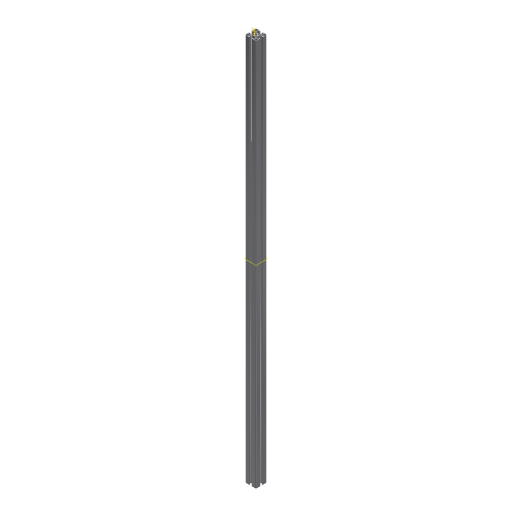
# Autodesk Inventor part: Profil-40x40x1200
Saved by Autodesk Inventor 2024.3 (Build 283343000, 343)
## iProperties
Created: 2012-07-12
Part Number: Profil-40x40x1200
Document SubType Name: Modeling
Designer: rd
Density: 2.7 g/cm^3
Material: Aluminium 6061
Appearance: Aluminium - poliert
Mass: 416.439 g
Surface Area: 1756.69 cm^2
Volume: 154.237 cm^3
Author: rd
Autodesk Inventor part; units mm, degrees
ref_plane "YZ Plane" through (0, 0, 0) normal (1, 0, 0) x (0, 1, 0)
ref_plane "XZ Plane" through (0, 0, 0) normal (0, 1, 0) x (-1, 0, 0)
sketch "Skizze1" plane through (0, 0, 0) normal (0, 0, 1) x (1, 0, 0)
  line L0 (4.8272, 8.2658) -> (6.2339, 9.6725)
  arc A0 (6.8957, 9.7126) -> (6.2339, 9.6725) centre (6.5874, 9.3189) ccw
  line L1 (6.8957, 9.7126) -> (7.2389, 9.4483)
  arc A1 (7.2389, 9.4483) -> (9.17, 8.8) centre (9.17, 12) ccw
  line L2 (9.17, 8.8) -> (12.7997, 8.8)
  arc A2 (13.2997, 8.3) -> (12.7997, 8.8) centre (12.7997, 8.3) ccw
  line L3 (13.2997, 8.3) -> (13.2997, 4)
  arc A3 (10.4997, 1.2) -> (13.2997, 4) centre (10.4997, 4) ccw
  line L4 (10.4997, 1.2) -> (6.1997, 1.2)
  arc A4 (5.6997, 1.7) -> (6.1997, 1.2) centre (6.1997, 1.7) ccw
  line L5 (5.6997, 1.7) -> (5.6997, 5.3296)
  arc A5 (5.6997, 5.3296) -> (5.0513, 7.2607) centre (2.4997, 5.3296) ccw
  line L6 (5.0513, 7.2607) -> (4.7871, 7.6039)
  arc A6 (4.8272, 8.2658) -> (4.7871, 7.6039) centre (5.1807, 7.9122) ccw
  line L7 (-15.8272, 31.7342) -> (-17.2339, 30.3275)
  arc A7 (-17.8957, 30.2874) -> (-17.2339, 30.3275) centre (-17.5874, 30.6811) ccw
  line L8 (-17.8957, 30.2874) -> (-18.2389, 30.5517)
  arc A8 (-18.2389, 30.5517) -> (-20.17, 31.2) centre (-20.17, 28) ccw
  line L9 (-20.17, 31.2) -> (-23.7997, 31.2)
  arc A9 (-24.2997, 31.7) -> (-23.7997, 31.2) centre (-23.7997, 31.7) ccw
  line L10 (-24.2997, 31.7) -> (-24.2997, 36)
  arc A10 (-21.4997, 38.8) -> (-24.2997, 36) centre (-21.4997, 36) ccw
  line L11 (-21.4997, 38.8) -> (-17.1997, 38.8)
  arc A11 (-16.6997, 38.3) -> (-17.1997, 38.8) centre (-17.1997, 38.3) ccw
  line L12 (-16.6997, 38.3) -> (-16.6997, 34.6704)
  arc A12 (-16.6997, 34.6704) -> (-16.0513, 32.7393) centre (-13.4997, 34.6704) ccw
  line L13 (-16.0513, 32.7393) -> (-15.7871, 32.3961)
  arc A13 (-15.8272, 31.7342) -> (-15.7871, 32.3961) centre (-16.1807, 32.0878) ccw
  line L14 (6.2342, 30.3272) -> (4.8275, 31.7339)
  arc A14 (4.7874, 32.3957) -> (4.8275, 31.7339) centre (5.1811, 32.0874) ccw
  line L15 (4.7874, 32.3957) -> (5.0517, 32.7389)
  arc A15 (5.0517, 32.7389) -> (5.7, 34.67) centre (2.5, 34.67) ccw
  line L16 (5.7, 34.67) -> (5.7, 38.2997)
  arc A16 (6.2, 38.7997) -> (5.7, 38.2997) centre (6.2, 38.2997) ccw
  line L17 (6.2, 38.7997) -> (10.5, 38.7997)
  arc A17 (13.3, 35.9997) -> (10.5, 38.7997) centre (10.5, 35.9997) ccw
  line L18 (13.3, 35.9997) -> (13.3, 31.6997)
  arc A18 (12.8, 31.1997) -> (13.3, 31.6997) centre (12.8, 31.6997) ccw
  line L19 (12.8, 31.1997) -> (9.1704, 31.1997)
  arc A19 (9.1704, 31.1997) -> (7.2393, 30.5513) centre (9.1704, 27.9997) ccw
  line L20 (7.2393, 30.5513) -> (6.8961, 30.2871)
  arc A20 (6.2342, 30.3272) -> (6.8961, 30.2871) centre (6.5878, 30.6807) ccw
  line L21 (-17.2342, 9.6728) -> (-15.8275, 8.2661)
  arc A21 (-15.7874, 7.6043) -> (-15.8275, 8.2661) centre (-16.1811, 7.9126) ccw
  line L22 (-15.7874, 7.6043) -> (-16.0517, 7.2611)
  arc A22 (-16.0517, 7.2611) -> (-16.7, 5.33) centre (-13.5, 5.33) ccw
  line L23 (-16.7, 5.33) -> (-16.7, 1.7003)
  arc A23 (-17.2, 1.2003) -> (-16.7, 1.7003) centre (-17.2, 1.7003) ccw
  line L24 (-17.2, 1.2003) -> (-21.5, 1.2003)
  arc A24 (-24.3, 4.0003) -> (-21.5, 1.2003) centre (-21.5, 4.0003) ccw
  line L25 (-24.3, 4.0003) -> (-24.3, 8.3003)
  arc A25 (-23.8, 8.8003) -> (-24.3, 8.3003) centre (-23.8, 8.3003) ccw
  line L26 (-23.8, 8.8003) -> (-20.1704, 8.8003)
  arc A26 (-20.1704, 8.8003) -> (-18.2393, 9.4487) centre (-20.1704, 12.0003) ccw
  line L27 (-18.2393, 9.4487) -> (-17.8961, 9.7129)
  arc A27 (-17.2342, 9.6728) -> (-17.8961, 9.7129) centre (-17.5878, 9.3193) ccw
  circle A28 centre (-5.5, 20) radius 3.4
  arc A29 (-8, 15.3902) -> (-8.2273, 15.8093) centre (-8.5, 15.3902) ccw
  line L28 (-8, 15.3902) -> (-8, 13.9018)
  arc A30 (-8.4351, 13.406) -> (-8, 13.9018) centre (-8.5, 13.9018) ccw
  arc A31 (-8.4351, 13.406) -> (-10.88, 12.41) centre (-7.76, 8.25) ccw
  arc A32 (-10.88, 12.41) -> (-14.3828, 9.2523) centre (4.84, -8.55) ccw
  arc A33 (-15.1032, 9.2385) -> (-14.3828, 9.2523) centre (-14.7497, 9.5921) ccw
  line L29 (-15.1032, 9.2385) -> (-16.2615, 10.3968)
  arc A34 (-16.2477, 11.1172) -> (-16.2615, 10.3968) centre (-15.9079, 10.7503) ccw
  arc A35 (-16.2477, 11.1172) -> (-13.09, 14.62) centre (-34.05, 30.34) ccw
  arc A36 (-13.09, 14.62) -> (-12.094, 17.0649) centre (-17.25, 17.74) ccw
  arc A37 (-11.5982, 17.5) -> (-12.094, 17.0649) centre (-11.5982, 17) ccw
  line L30 (-11.5982, 17.5) -> (-10.1098, 17.5)
  arc A38 (-9.6907, 17.2727) -> (-10.1098, 17.5) centre (-10.1098, 17) ccw
  arc A39 (-9.6907, 17.2727) -> (-8.2273, 15.8093) centre (-5.5, 20) ccw
  arc A40 (-3, 24.6098) -> (-2.7727, 24.1907) centre (-2.5, 24.6098) ccw
  line L31 (-3, 24.6098) -> (-3, 26.0982)
  arc A41 (-2.5649, 26.594) -> (-3, 26.0982) centre (-2.5, 26.0982) ccw
  arc A42 (-2.5649, 26.594) -> (-0.12, 27.59) centre (-3.24, 31.75) ccw
  arc A43 (-0.12, 27.59) -> (3.3828, 30.7477) centre (-15.84, 48.55) ccw
  arc A44 (4.1032, 30.7615) -> (3.3828, 30.7477) centre (3.7497, 30.4079) ccw
  line L32 (4.1032, 30.7615) -> (5.2615, 29.6032)
  arc A45 (5.2477, 28.8828) -> (5.2615, 29.6032) centre (4.9079, 29.2497) ccw
  arc A46 (5.2477, 28.8828) -> (2.09, 25.38) centre (23.05, 9.66) ccw
  arc A47 (2.09, 25.38) -> (1.094, 22.9351) centre (6.25, 22.26) ccw
  arc A48 (0.5982, 22.5) -> (1.094, 22.9351) centre (0.5982, 23) ccw
  line L33 (0.5982, 22.5) -> (-0.8902, 22.5)
  arc A49 (-1.3093, 22.7273) -> (-0.8902, 22.5) centre (-0.8902, 23) ccw
  arc A50 (-1.3093, 22.7273) -> (-2.7727, 24.1907) centre (-5.5, 20) ccw
  arc A51 (-0.8902, 17.5) -> (-1.3093, 17.2727) centre (-0.8902, 17) ccw
  line L34 (-0.8902, 17.5) -> (0.5982, 17.5)
  arc A52 (1.094, 17.0649) -> (0.5982, 17.5) centre (0.5982, 17) ccw
  arc A53 (1.094, 17.0649) -> (2.09, 14.62) centre (6.25, 17.74) ccw
  arc A54 (2.09, 14.62) -> (5.2477, 11.1172) centre (23.05, 30.34) ccw
  arc A55 (5.2615, 10.3968) -> (5.2477, 11.1172) centre (4.9079, 10.7503) ccw
  line L35 (5.2615, 10.3968) -> (4.1032, 9.2385)
  arc A56 (3.3828, 9.2523) -> (4.1032, 9.2385) centre (3.7497, 9.5921) ccw
  arc A57 (3.3828, 9.2523) -> (-0.12, 12.41) centre (-15.84, -8.55) ccw
  arc A58 (-0.12, 12.41) -> (-2.5649, 13.406) centre (-3.24, 8.25) ccw
  arc A59 (-3, 13.9018) -> (-2.5649, 13.406) centre (-2.5, 13.9018) ccw
  line L36 (-3, 13.9018) -> (-3, 15.3902)
  arc A60 (-2.7727, 15.8093) -> (-3, 15.3902) centre (-2.5, 15.3902) ccw
  arc A61 (-2.7727, 15.8093) -> (-1.3093, 17.2727) centre (-5.5, 20) ccw
  arc A62 (-10.1098, 22.5) -> (-9.6907, 22.7273) centre (-10.1098, 23) ccw
  line L37 (-10.1098, 22.5) -> (-11.5982, 22.5)
  arc A63 (-12.094, 22.9351) -> (-11.5982, 22.5) centre (-11.5982, 23) ccw
  arc A64 (-12.094, 22.9351) -> (-13.09, 25.38) centre (-17.25, 22.26) ccw
  arc A65 (-13.09, 25.38) -> (-16.2477, 28.8828) centre (-34.05, 9.66) ccw
  arc A66 (-16.2615, 29.6032) -> (-16.2477, 28.8828) centre (-15.9079, 29.2497) ccw
  line L38 (-16.2615, 29.6032) -> (-15.1032, 30.7615)
  arc A67 (-14.3828, 30.7477) -> (-15.1032, 30.7615) centre (-14.7497, 30.4079) ccw
  arc A68 (-14.3828, 30.7477) -> (-10.88, 27.59) centre (4.84, 48.55) ccw
  arc A69 (-10.88, 27.59) -> (-8.4351, 26.594) centre (-7.76, 31.75) ccw
  arc A70 (-8, 26.0982) -> (-8.4351, 26.594) centre (-8.5, 26.0982) ccw
  line L39 (-8, 26.0982) -> (-8, 24.6098)
  arc A71 (-8.2273, 24.1907) -> (-8, 24.6098) centre (-8.5, 24.6098) ccw
  arc A72 (-8.2273, 24.1907) -> (-9.6907, 22.7273) centre (-5.5, 20) ccw
  line L40 (-1.5, 1.5) -> (-1.5, 3.5)
  arc A73 (-1.5, 1.5) -> (0, 0) centre (0, 1.5) ccw
  line L41 (10.5, 0) -> (0, 0)
  arc A74 (10.5, 0) -> (14.5, 4) centre (10.5, 4) ccw
  line L42 (14.5, 14.5) -> (14.5, 4)
  arc A75 (14.5, 14.5) -> (13, 16) centre (13, 14.5) ccw
  line L43 (11, 16) -> (13, 16)
  arc A76 (11, 16) -> (10, 15) centre (11, 15) ccw
  line L44 (10, 13.25) -> (10, 15)
  arc A77 (10, 13.25) -> (10.25, 13) centre (10.25, 13.25) ccw
  line L45 (12.25, 13) -> (10.25, 13)
  arc A78 (12.5, 12.75) -> (12.25, 13) centre (12.25, 12.75) ccw
  line L46 (12.5, 12.5) -> (12.5, 12.75)
  arc A79 (10, 10) -> (12.5, 12.5) centre (10, 12.5) ccw
  line L47 (9.2204, 10) -> (10, 10)
  arc A80 (8.0134, 10.4052) -> (9.2204, 10) centre (9.2204, 12) ccw
  arc A81 (3.0405, 15.4197) -> (8.0134, 10.4052) centre (23.1, 30.34) ccw
  arc A82 (2.25, 17.8069) -> (3.0405, 15.4197) centre (6.25, 17.8069) ccw
  line L48 (2.25, 22.1931) -> (2.25, 17.8069)
  arc A83 (3.0405, 24.5803) -> (2.25, 22.1931) centre (6.25, 22.1931) ccw
  arc A84 (8.0134, 29.5948) -> (3.0405, 24.5803) centre (23.1, 9.66) ccw
  arc A85 (9.2204, 30) -> (8.0134, 29.5948) centre (9.2204, 28) ccw
  line L49 (10, 30) -> (9.2204, 30)
  arc A86 (12.5, 27.5) -> (10, 30) centre (10, 27.5) ccw
  line L50 (12.5, 27.25) -> (12.5, 27.5)
  arc A87 (12.25, 27) -> (12.5, 27.25) centre (12.25, 27.25) ccw
  line L51 (10.25, 27) -> (12.25, 27)
  arc A88 (10.25, 27) -> (10, 26.75) centre (10.25, 26.75) ccw
  line L52 (10, 25) -> (10, 26.75)
  arc A89 (10, 25) -> (11, 24) centre (11, 25) ccw
  line L53 (13, 24) -> (11, 24)
  arc A90 (13, 24) -> (14.5, 25.5) centre (13, 25.5) ccw
  line L54 (14.5, 36) -> (14.5, 25.5)
  arc A91 (14.5, 36) -> (10.5, 40) centre (10.5, 36) ccw
  line L55 (0, 40) -> (10.5, 40)
  arc A92 (0, 40) -> (-1.5, 38.5) centre (0, 38.5) ccw
  line L56 (-1.5, 36.5) -> (-1.5, 38.5)
  arc A93 (-1.5, 36.5) -> (-0.5, 35.5) centre (-0.5, 36.5) ccw
  line L57 (1.25, 35.5) -> (-0.5, 35.5)
  arc A94 (1.25, 35.5) -> (1.5, 35.75) centre (1.25, 35.75) ccw
  line L58 (1.5, 37.75) -> (1.5, 35.75)
  arc A95 (1.75, 38) -> (1.5, 37.75) centre (1.75, 37.75) ccw
  line L59 (2, 38) -> (1.75, 38)
  arc A96 (4.5, 35.5) -> (2, 38) centre (2, 35.5) ccw
  line L60 (4.5, 34.7204) -> (4.5, 35.5)
  arc A97 (4.0948, 33.5134) -> (4.5, 34.7204) centre (2.5, 34.7204) ccw
  arc A98 (-0.9197, 28.5405) -> (4.0948, 33.5134) centre (-15.84, 48.6) ccw
  arc A99 (-3.3069, 27.75) -> (-0.9197, 28.5405) centre (-3.3069, 31.75) ccw
  line L61 (-7.6931, 27.75) -> (-3.3069, 27.75)
  arc A100 (-10.0803, 28.5405) -> (-7.6931, 27.75) centre (-7.6931, 31.75) ccw
  arc A101 (-15.0948, 33.5134) -> (-10.0803, 28.5405) centre (4.84, 48.6) ccw
  arc A102 (-15.5, 34.7204) -> (-15.0948, 33.5134) centre (-13.5, 34.7204) ccw
  line L62 (-15.5, 35.5) -> (-15.5, 34.7204)
  arc A103 (-13, 38) -> (-15.5, 35.5) centre (-13, 35.5) ccw
  line L63 (-12.75, 38) -> (-13, 38)
  arc A104 (-12.5, 37.75) -> (-12.75, 38) centre (-12.75, 37.75) ccw
  line L64 (-12.5, 35.75) -> (-12.5, 37.75)
  arc A105 (-12.5, 35.75) -> (-12.25, 35.5) centre (-12.25, 35.75) ccw
  line L65 (-10.5, 35.5) -> (-12.25, 35.5)
  arc A106 (-10.5, 35.5) -> (-9.5, 36.5) centre (-10.5, 36.5) ccw
  line L66 (-9.5, 38.5) -> (-9.5, 36.5)
  arc A107 (-9.5, 38.5) -> (-11, 40) centre (-11, 38.5) ccw
  line L67 (-21.5, 40) -> (-11, 40)
  arc A108 (-21.5, 40) -> (-25.5, 36) centre (-21.5, 36) ccw
  line L68 (-25.5, 25.5) -> (-25.5, 36)
  arc A109 (-25.5, 25.5) -> (-24, 24) centre (-24, 25.5) ccw
  line L69 (-22, 24) -> (-24, 24)
  arc A110 (-22, 24) -> (-21, 25) centre (-22, 25) ccw
  line L70 (-21, 26.75) -> (-21, 25)
  arc A111 (-21, 26.75) -> (-21.25, 27) centre (-21.25, 26.75) ccw
  line L71 (-23.25, 27) -> (-21.25, 27)
  arc A112 (-23.5, 27.25) -> (-23.25, 27) centre (-23.25, 27.25) ccw
  line L72 (-23.5, 27.5) -> (-23.5, 27.25)
  arc A113 (-21, 30) -> (-23.5, 27.5) centre (-21, 27.5) ccw
  line L73 (-20.2204, 30) -> (-21, 30)
  arc A114 (-19.0134, 29.5948) -> (-20.2204, 30) centre (-20.2204, 28) ccw
  arc A115 (-14.0405, 24.5803) -> (-19.0134, 29.5948) centre (-34.1, 9.66) ccw
  arc A116 (-13.25, 22.1931) -> (-14.0405, 24.5803) centre (-17.25, 22.1931) ccw
  line L74 (-13.25, 17.8069) -> (-13.25, 22.1931)
  arc A117 (-14.0405, 15.4197) -> (-13.25, 17.8069) centre (-17.25, 17.8069) ccw
  arc A118 (-19.0134, 10.4052) -> (-14.0405, 15.4197) centre (-34.1, 30.34) ccw
  arc A119 (-20.2204, 10) -> (-19.0134, 10.4052) centre (-20.2204, 12) ccw
  line L75 (-21, 10) -> (-20.2204, 10)
  arc A120 (-23.5, 12.5) -> (-21, 10) centre (-21, 12.5) ccw
  line L76 (-23.5, 12.75) -> (-23.5, 12.5)
  arc A121 (-23.25, 13) -> (-23.5, 12.75) centre (-23.25, 12.75) ccw
  line L77 (-21.25, 13) -> (-23.25, 13)
  arc A122 (-21.25, 13) -> (-21, 13.25) centre (-21.25, 13.25) ccw
  line L78 (-21, 15) -> (-21, 13.25)
  arc A123 (-21, 15) -> (-22, 16) centre (-22, 15) ccw
  line L79 (-24, 16) -> (-22, 16)
  arc A124 (-24, 16) -> (-25.5, 14.5) centre (-24, 14.5) ccw
  line L80 (-25.5, 4) -> (-25.5, 14.5)
  arc A125 (-25.5, 4) -> (-21.5, 0) centre (-21.5, 4) ccw
  line L81 (-11, 0) -> (-21.5, 0)
  arc A126 (-11, 0) -> (-9.5, 1.5) centre (-11, 1.5) ccw
  line L82 (-9.5, 3.5) -> (-9.5, 1.5)
  arc A127 (-9.5, 3.5) -> (-10.5, 4.5) centre (-10.5, 3.5) ccw
  line L83 (-12.25, 4.5) -> (-10.5, 4.5)
  arc A128 (-12.25, 4.5) -> (-12.5, 4.25) centre (-12.25, 4.25) ccw
  line L84 (-12.5, 2.25) -> (-12.5, 4.25)
  arc A129 (-12.75, 2) -> (-12.5, 2.25) centre (-12.75, 2.25) ccw
  line L85 (-13, 2) -> (-12.75, 2)
  arc A130 (-15.5, 4.5) -> (-13, 2) centre (-13, 4.5) ccw
  line L86 (-15.5, 5.2796) -> (-15.5, 4.5)
  arc A131 (-15.0948, 6.4866) -> (-15.5, 5.2796) centre (-13.5, 5.2796) ccw
  arc A132 (-10.0803, 11.4595) -> (-15.0948, 6.4866) centre (4.84, -8.6) ccw
  arc A133 (-7.6931, 12.25) -> (-10.0803, 11.4595) centre (-7.6931, 8.25) ccw
  line L87 (-3.3069, 12.25) -> (-7.6931, 12.25)
  arc A134 (-0.9197, 11.4595) -> (-3.3069, 12.25) centre (-3.3069, 8.25) ccw
  arc A135 (4.0948, 6.4866) -> (-0.9197, 11.4595) centre (-15.84, -8.6) ccw
  arc A136 (4.5, 5.2796) -> (4.0948, 6.4866) centre (2.5, 5.2796) ccw
  line L88 (4.5, 4.5) -> (4.5, 5.2796)
  arc A137 (2, 2) -> (4.5, 4.5) centre (2, 4.5) ccw
  line L89 (1.75, 2) -> (2, 2)
  arc A138 (1.5, 2.25) -> (1.75, 2) centre (1.75, 2.25) ccw
  line L90 (1.5, 4.25) -> (1.5, 2.25)
  arc A139 (1.5, 4.25) -> (1.25, 4.5) centre (1.25, 4.25) ccw
  line L91 (-0.5, 4.5) -> (1.25, 4.5)
  arc A140 (-0.5, 4.5) -> (-1.5, 3.5) centre (-0.5, 3.5) ccw
  point P0 (0, 0)
  point P1 (-25.5, 0)
  constraints: 280 point on circle, 184 end point, 141 centre point
extrude "Extrusion1" add sketch "Skizze1" along normal mid plane 1400
ref_plane "Arbeitsebene1" through (-21.5, 20, 700) normal (0, -1, 0) x (1, 0, 0)
ref_plane "Arbeitsebene2" through (-5.5, 4, 700) normal (1, 0, 0) x (0, 0, -1)
